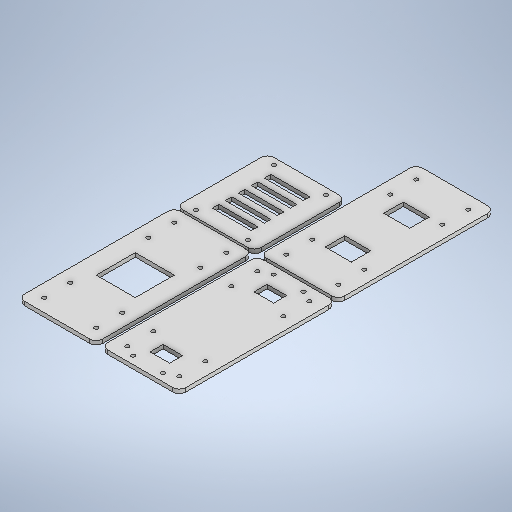
# Autodesk Inventor part: Pieza1
Saved by Autodesk Inventor 2025.2 (Build 292293000, 293)
## iProperties
Created: 2025-02-14
Part Number: Pieza1
Material: Genérico
Document SubType Name: Modeling
Designer: alex
Density: 1 g/cm^3
Appearance: Valor por defecto
Author: alex
Autodesk Inventor part; units mm, degrees
ref_plane "YZ Plane" through (0, 0, 0) normal (1, 0, 0) x (0, 1, 0)
ref_plane "XZ Plane" through (0, 0, 0) normal (0, 1, 0) x (-1, 0, 0)
ref_plane "XY Plane" through (0, 0, 0) normal (0, 0, 1) x (1, 0, 0)
sketch "Boceto1" plane through (0, 0, 0) normal (0, 1, 0) x (-1, 0, 0)
  line L0 (5, 0) -> (55, 0)
  line L1 (60, -5) -> (60, -115)
  line L2 (55, -120) -> (5, -120)
  line L3 (0, -115) -> (0, -5)
  line L4 (37.5, -95) -> (22.5, -95)
  line L5 (22.5, -95) -> (22.5, -105)
  line L6 (22.5, -105) -> (37.5, -105)
  line L7 (37.5, -105) -> (37.5, -95)
  circle A0 centre (50, -10) radius 1.5
  line L8 (37.5, -15) -> (22.5, -15)
  line L9 (22.5, -15) -> (22.5, -25)
  line L10 (22.5, -25) -> (37.5, -25)
  line L11 (37.5, -25) -> (37.5, -15)
  circle A1 centre (10, -10) radius 1.5
  circle A2 centre (10, -110) radius 1.5
  circle A3 centre (50, -110) radius 1.5
  line L12 (69.3189, -0.4209) -> (119.3189, -0.4209)
  line L13 (124.3189, -5.4209) -> (124.3189, -115.4209)
  line L14 (119.3189, -120.4209) -> (69.3189, -120.4209)
  line L15 (64.3189, -115.4209) -> (64.3189, -5.4209)
  circle A4 centre (114.3189, -10.4209) radius 1.5
  circle A5 centre (74.3189, -10.4209) radius 1.5
  circle A6 centre (74.3189, -110.4209) radius 1.5
  circle A7 centre (114.3189, -110.4209) radius 1.5
  circle A8 centre (114.3189, -30.4209) radius 1.5
  circle A9 centre (74.3189, -30.4209) radius 1.5
  circle A10 centre (114.3189, -90.4209) radius 1.5
  circle A11 centre (74.3189, -90.4209) radius 1.5
  line L16 (109.3189, -45.4209) -> (79.3189, -45.4209)
  line L17 (79.3189, -45.4209) -> (79.3189, -75.4209)
  line L18 (79.3189, -75.4209) -> (109.3189, -75.4209)
  line L19 (109.3189, -75.4209) -> (109.3189, -45.4209)
  arc A12 (60, -5) -> (55, 0) centre (55, -5) ccw
  arc A13 (5, 0) -> (0, -5) centre (5, -5) ccw
  arc A14 (0, -115) -> (5, -120) centre (5, -115) ccw
  arc A15 (55, -120) -> (60, -115) centre (55, -115) ccw
  arc A16 (69.3189, -0.4209) -> (64.3189, -5.4209) centre (69.3189, -5.4209) ccw
  arc A17 (124.3189, -5.4209) -> (119.3189, -0.4209) centre (119.3189, -5.4209) ccw
  arc A18 (119.3189, -120.4209) -> (124.3189, -115.4209) centre (119.3189, -115.4209) ccw
  arc A19 (64.3189, -115.4209) -> (69.3189, -120.4209) centre (69.3189, -115.4209) ccw
  circle A20 centre (50, -30) radius 1.5
  circle A21 centre (50, -90) radius 1.5
  circle A22 centre (10, -30) radius 1.5
  circle A23 centre (10, -90) radius 1.5
  circle A24 centre (49.9595, -232.1797) radius 1.5
  circle A25 centre (9.9595, -232.1797) radius 1.5
  line L20 (54.9595, -242.1797) -> (4.9595, -242.1797)
  line L21 (59.9595, -127.1797) -> (59.9595, -237.1797)
  line L22 (-0.0405, -237.1797) -> (-0.0405, -127.1797)
  circle A26 centre (9.9595, -132.1797) radius 1.5
  line L23 (4.9595, -122.1797) -> (54.9595, -122.1797)
  circle A27 centre (49.9595, -132.1797) radius 1.5
  circle A28 centre (49.9595, -152.1797) radius 1.5
  circle A29 centre (9.9595, -152.1797) radius 1.5
  circle A30 centre (49.9595, -212.1797) radius 1.5
  circle A31 centre (9.9595, -212.1797) radius 1.5
  line L24 (39.9595, -152.1797) -> (19.9595, -152.1797)
  line L25 (19.9595, -152.1797) -> (19.9595, -167.1797)
  line L26 (19.9595, -167.1797) -> (39.9595, -167.1797)
  line L27 (39.9595, -167.1797) -> (39.9595, -152.1797)
  arc A32 (4.9595, -122.1797) -> (-0.0405, -127.1797) centre (4.9595, -127.1797) ccw
  arc A33 (59.9595, -127.1797) -> (54.9595, -122.1797) centre (54.9595, -127.1797) ccw
  arc A34 (54.9595, -242.1797) -> (59.9595, -237.1797) centre (54.9595, -237.1797) ccw
  arc A35 (-0.0405, -237.1797) -> (4.9595, -242.1797) centre (4.9595, -237.1797) ccw
  line L28 (39.9595, -212.1797) -> (39.9595, -197.1797)
  line L29 (39.9595, -197.1797) -> (19.9595, -197.1797)
  line L30 (19.9595, -197.1797) -> (19.9595, -212.1797)
  line L31 (19.9595, -212.1797) -> (39.9595, -212.1797)
  line L32 (119.3189, -122.1797) -> (69.3189, -122.1797)
  line L33 (64.3189, -127.1797) -> (64.3189, -187.1797)
  line L34 (69.3189, -192.1797) -> (119.3189, -192.1797)
  line L35 (124.3189, -187.1797) -> (124.3189, -127.1797)
  circle A36 centre (114.3189, -127.1797) radius 1.5
  circle A37 centre (74.3189, -127.1797) radius 1.5
  circle A38 centre (74.3189, -187.1797) radius 1.5
  circle A39 centre (114.3189, -187.1797) radius 1.5
  arc A40 (69.3189, -122.1797) -> (64.3189, -127.1797) centre (69.3189, -127.1797) ccw
  arc A41 (124.3189, -127.1797) -> (119.3189, -122.1797) centre (119.3189, -127.1797) ccw
  arc A42 (119.3189, -192.1797) -> (124.3189, -187.1797) centre (119.3189, -187.1797) ccw
  arc A43 (64.3189, -187.1797) -> (69.3189, -192.1797) centre (69.3189, -187.1797) ccw
  line L36 (109.3189, -134.6797) -> (79.3189, -134.6797)
  line L37 (79.3189, -134.6797) -> (79.3189, -139.6797)
  line L38 (79.3189, -139.6797) -> (109.3189, -139.6797)
  line L39 (109.3189, -139.6797) -> (109.3189, -134.6797)
  line L40 (109.3189, -154.6797) -> (79.3189, -154.6797)
  line L41 (79.3189, -154.6797) -> (79.3189, -159.6797)
  line L42 (79.3189, -159.6797) -> (109.3189, -159.6797)
  line L43 (109.3189, -159.6797) -> (109.3189, -154.6797)
  line L44 (109.3189, -174.6797) -> (79.3189, -174.6797)
  line L45 (79.3189, -174.6797) -> (79.3189, -179.6797)
  line L46 (79.3189, -179.6797) -> (109.3189, -179.6797)
  line L47 (109.3189, -179.6797) -> (109.3189, -174.6797)
  line L48 (109.3189, -144.6797) -> (79.3189, -144.6797)
  line L49 (79.3189, -144.6797) -> (79.3189, -149.6797)
  line L50 (79.3189, -149.6797) -> (109.3189, -149.6797)
  line L51 (109.3189, -149.6797) -> (109.3189, -144.6797)
  line L52 (109.3189, -164.6797) -> (79.3189, -164.6797)
  line L53 (79.3189, -164.6797) -> (79.3189, -169.6797)
  line L54 (79.3189, -169.6797) -> (109.3189, -169.6797)
  line L55 (109.3189, -169.6797) -> (109.3189, -164.6797)
  point P0 (0, 0)
  point P1 (60, -120)
  point P2 (60, 0)
  point P3 (0, -120)
  point P4 (22.5, -100)
  point P5 (22.5, -20)
  point P6 (30, -15)
  point P7 (124.3189, -120.4209)
  point P8 (124.3189, -0.4209)
  point P9 (64.3189, -120.4209)
  point P10 (94.3189, -0.4209)
  point P11 (94.3189, -45.4209)
  point P12 (59.9595, -242.1797)
  point P13 (-0.0405, -242.1797)
  point P14 (59.9595, -122.1797)
  point P15 (29.9595, -122.1797)
  point P16 (29.9595, -152.1797)
  point P17 (29.9595, -197.1797)
  point P18 (29.9595, -212.1797)
  point P19 (79.3189, -147.1797)
  point P20 (79.3189, -167.1797)
  dimension "d0" = 60
  dimension "d1" = 120
  dimension "d2" = 15
  dimension "d3" = 10
  dimension "d4" = 3
  dimension "d5" = 15
  dimension "d6" = 22.5
  dimension "d7" = 15
  dimension "d8" = 10
  dimension "d9" = 3
  dimension "d10" = 3
  dimension "d11" = 3
  dimension "d12" = 22.5
  dimension "d13" = 15
  dimension "d14" = 10
  dimension "d15" = 10
  dimension "d16" = 10
  dimension "d17" = 10
  dimension "d18" = 10
  dimension "d19" = 10
  dimension "d20" = 10
  dimension "d21" = 10
  dimension "d22" = 60
  dimension "d23" = 120
  dimension "d26" = 3
  dimension "d32" = 3
  dimension "d33" = 3
  dimension "d36" = 10
  dimension "d37" = 10
  dimension "d39" = 10
  dimension "d40" = 10
  dimension "d41" = 10
  dimension "d42" = 10
  dimension "d43" = 10
  dimension "d44" = 3
  dimension "d45" = 3
  dimension "d46" = 3
  dimension "d47" = 3
  dimension "d48" = 10
  dimension "d49" = 10
  dimension "d50" = 10
  dimension "d51" = 10
  dimension "d52" = 60
  dimension "d53" = 30
  dimension "d54" = 60
  dimension "d55" = 30
  dimension "d56" = 30
  dimension "d57" = 30
  dimension "d58" = 45
  dimension "d59" = 5
  dimension "d60" = 5
  dimension "d61" = 5
  dimension "d62" = 5
  dimension "d63" = 3
  dimension "d64" = 3
  dimension "d65" = 3
  dimension "d66" = 3
  dimension "d67" = 10
  dimension "d68" = 10
  dimension "d69" = 10
  dimension "d70" = 10
  dimension "d71" = 30
  dimension "d72" = 30
  dimension "d73" = 30
  constraints: 112 end point, 44 centre point, 32 point on circle, 32 tangent, 28 parallel, 20 point on line, 14 horizontal, 14 perpendicular, 11 midpoint, 10 equal radius
  measures "d0" distance of point (60, -120) point (0, -120)
  measures "d1" distance of point (60, 0) point (60, -120)
  measures "d2" distance of L6.end L5.end
  measures "d3" distance of L5.end L4.end
  measures "d4" diameter of A0
  measures "d5" distance between parallel lines of L2 L6
  measures "d6" distance from line of L3 point (22.5, -100)
  measures "d7" distance of L10.end L9.end
  measures "d8" distance of L9.end L8.end
  measures "d9" diameter of A1
  measures "d10" diameter of A2
  measures "d11" diameter of A3
  measures "d12" distance between parallel lines of L3 L9
  measures "d13" distance from line of L0 point (30, -15)
  measures "d14" distance from line of L0 A0.centre
  measures "d15" distance from line of L1 A0.centre
  measures "d16" distance from line of L0 A1.centre
  measures "d17" distance from line of L3 A1.centre
  measures "d18" distance from line of L2 A3.centre
  measures "d19" distance from line of L1 A3.centre
  measures "d20" distance from line of L2 A2.centre
  measures "d21" distance from line of L3 A2.centre
  measures "d22" distance of point (124.319, -120.421) point (64.319, -120.421)
  measures "d23" distance of point (124.319, -0.421) point (124.319, -120.421)
  measures "d26" diameter of A4
  measures "d32" diameter of A6
  measures "d33" diameter of A7
  measures "d36" distance from line of L12 A4.centre
  measures "d37" distance from line of L13 A4.centre
  measures "d39" distance from line of L15 A5.centre
  measures "d40" distance from line of L14 A7.centre
  measures "d41" distance from line of L13 A7.centre
  measures "d42" distance from line of L14 A6.centre
  measures "d43" distance from line of L15 A6.centre
  measures "d44" diameter of A8
  measures "d45" diameter of A9
  measures "d46" diameter of A10
  measures "d47" diameter of A11
  measures "d48" distance from line of L13 A8.centre
  measures "d49" distance from line of L13 A10.centre
  measures "d50" distance from line of L15 A9.centre
  measures "d51" distance from line of L15 A11.centre
  measures "d52" distance of A10.centre A8.centre
  measures "d53" distance from line of L12 A8.centre
  measures "d54" distance of A11.centre A9.centre
  measures "d55" distance from line of L12 A9.centre
  measures "d56" distance of L17.end L18.end
  measures "d57" distance of L16.end L17.end
  measures "d58" distance of point (94.319, -0.421) point (94.319, -45.421)
  measures "d59" radius of A12
  measures "d60" radius of A13
  measures "d61" radius of A14
  measures "d62" radius of A15
  measures "d63" diameter of A20
  measures "d64" diameter of A21
  measures "d65" diameter of A22
  measures "d66" diameter of A23
  measures "d67" distance from line of L3 A23.centre
  measures "d68" distance from line of L3 A22.centre
  measures "d69" distance from line of L1 A21.centre
  measures "d70" distance from line of L1 A20.centre
  measures "d71" distance from line of L2 A21.centre
  measures "d72" distance from line of L0 A20.centre
  measures "d73" distance from line of L0 A22.centre
extrude "Extrusión1" add sketch "Boceto1" along normal blind 3
sketch "Boceto2" plane through (0, 3, 0) normal (0, 1, 0) x (1, 0, 0)
  circle A0 centre (-41.5, 6) radius 1.5
  circle A1 centre (-18.5, 6) radius 1.5
  line L0 (-55, 0) -> (-5, 0) projected
  line L1 (0, 5) -> (0, 115) projected
  line L2 (-60, 115) -> (-60, 5) projected
  circle A2 centre (-41.5, 114) radius 1.5
  circle A3 centre (-18.5, 114) radius 1.5
  line L3 (-5, 120) -> (-55, 120) projected
  point P0 (0, 0)
  dimension "d147" = 3
  dimension "d148" = 3
  dimension "d151" = 20
  dimension "d152" = 6
  dimension "d153" = 6
  dimension "d154" = 18.5
  dimension "d155" = 18.5
  dimension "d156" = 3
  dimension "d157" = 3
  dimension "d158" = 20
  dimension "d161" = 6
  dimension "d162" = 6
  dimension "d163" = 18.5
  constraints: 4 centre point
  measures "d147" diameter of A0
  measures "d148" diameter of A1
  measures "d152" distance from line of L0 A1.centre
  measures "d153" distance from line of A0.centre L0
  measures "d154" distance from line of L1 A1.centre
  measures "d155" distance from line of L2 A0.centre
  measures "d156" diameter of A2
  measures "d157" diameter of A3
  measures "d161" distance from line of L3 A2.centre
  measures "d162" distance from line of L3 A3.centre
  measures "d163" distance from line of L1 A3.centre
extrude "Extrusión2" cut sketch "Boceto2" against normal blind 3
